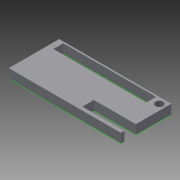
# Autodesk Inventor part: spi backpack model
Saved by Autodesk Inventor 2014 (Build 180170000, 170)
## iProperties
Created: 2014-07-20
Part Number: spi backpack model
Material: Generic
Document SubType Name: Modeling
Designer: james
Density: 1 g/cm^3
Appearance: Default
Author: james
Autodesk Inventor part; units mm, degrees
ref_plane "YZ Plane" through (0, 0, 0) normal (1, 0, 0) x (0, 1, 0)
ref_plane "XZ Plane" through (0, 0, 0) normal (0, 1, 0) x (-1, 0, 0)
ref_plane "XY Plane" through (0, 0, 0) normal (0, 0, 1) x (1, 0, 0)
sketch "Sketch1" plane through (0, 0, 0) normal (0, 0, 1) x (1, 0, 0)
  line L0 (32.6853, -22.1423) -> (32.6853, -16.9838)
  line L1 (32.6853, -16.9838) -> (51.489, -16.9838)
  line L2 (51.489, -16.9838) -> (51.489, -1.0089)
  line L3 (51.489, -1.0089) -> (1.0684, -1.0089)
  line L4 (1.0684, -1.0089) -> (1.0684, -23.6677)
  line L5 (1.0684, -23.6677) -> (51.489, -23.6677)
  line L6 (51.489, -23.6677) -> (51.489, -22.1423)
  line L7 (51.489, -22.1423) -> (32.6853, -22.1423)
  spline S0 degree 3 poles (48.8756, -2.4759) (49.6244, -2.4759) (50.2314, -3.0829) (50.2314, -3.8317) (50.2314, -4.5805) (49.6244, -5.1875) (48.8756, -5.1875) (48.1268, -5.1875) (47.5198, -4.5805) (47.5198, -3.8317) (47.5198, -3.0829) (48.1268, -2.4759) (48.8756, -2.4759) knots 0 0 0 0 1 1 1 2 2 2 3 3 3 4 4 4 4
  line L8 (48.8756, -2.4759) -> (49.6244, -2.4759) construction
  line L9 (49.6244, -2.4759) -> (50.2314, -3.0829) construction
  line L10 (50.2314, -3.0829) -> (50.2314, -3.8317) construction
  line L11 (50.2314, -3.8317) -> (50.2314, -4.5805) construction
  line L12 (50.2314, -4.5805) -> (49.6244, -5.1875) construction
  line L13 (49.6244, -5.1875) -> (48.8756, -5.1875) construction
  line L14 (48.8756, -5.1875) -> (48.1268, -5.1875) construction
  line L15 (48.1268, -5.1875) -> (47.5198, -4.5805) construction
  line L16 (47.5198, -4.5805) -> (47.5198, -3.8317) construction
  line L17 (47.5198, -3.8317) -> (47.5198, -3.0829) construction
  line L18 (47.5198, -3.0829) -> (48.1268, -2.4759) construction
  line L19 (48.1268, -2.4759) -> (48.8756, -2.4759) construction
  line L20 (3.6754, -1.73) -> (45.3598, -1.73)
  line L21 (45.3598, -1.73) -> (45.3598, -6.1952)
  line L22 (45.3598, -6.1952) -> (3.6754, -6.1952)
  line L23 (3.6754, -6.1952) -> (3.6754, -1.73)
  point P0 (0, 0)
  constraints: 24 end point, 2 other
sketch "Sketch3" plane through (0, 0, 0) normal (0, 0, 1) x (1, 0, 0)
  line L0 (51.4974, -22.1263) -> (51.4974, -23.7266)
  line L1 (51.4974, -23.7266) -> (1.1042, -23.7266)
  line L2 (1.1042, -23.7266) -> (1.1042, -1.0728)
  line L3 (1.1042, -1.0728) -> (51.4974, -1.0728)
  line L4 (51.4974, -1.0728) -> (51.4974, -17.0052)
  line L5 (51.4974, -17.0052) -> (32.6489, -17.0052)
  line L6 (32.6489, -17.0052) -> (32.6489, -22.1263)
  line L7 (32.6489, -22.1263) -> (51.4974, -22.1263)
  line L8 (3.7003, -1.7841) -> (45.3805, -1.7841)
  line L9 (45.3805, -1.7841) -> (45.3805, -6.2295)
  line L10 (45.3805, -6.2295) -> (3.7003, -6.2295)
  line L11 (3.7003, -6.2295) -> (3.7003, -1.7841)
  circle A0 centre (48.8657, -3.8112) radius 1.75
  point P0 (0, 0)
  dimension "d0" = 3.5
  constraints: 24 end point, 6 parallel, 3 perpendicular, 1 centre point, 1 collinear, 1 horizontal, 1 vertical
  measures "d0" diameter of A0
extrude "Extrusion1" add sketch "Sketch3" along normal blind 4.25
body "Solid1"
